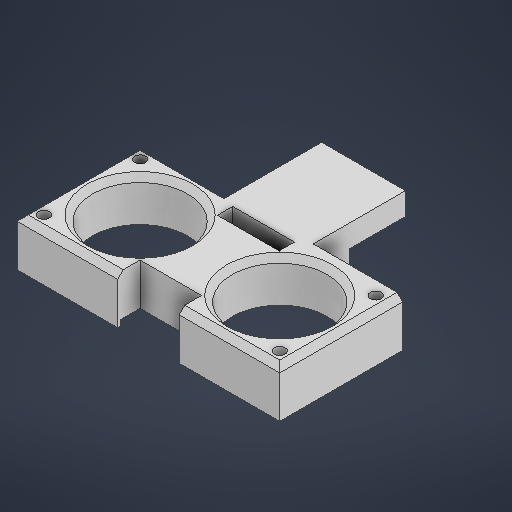
# Autodesk Inventor part: us-sensor-mount
Saved by Autodesk Inventor 2026.2 (Build 302298010, 298A)
## iProperties
Created: 2026-02-26
Part Number: us-sensor-mount
Material: Generic
Document SubType Name: Modeling
Designer: dm2166
Density: 1 g/cm^3
Appearance: Default
Author: dm2166
Autodesk Inventor part; units mm, degrees
ref_plane "YZ Plane" through (0, 0, 0) normal (1, 0, 0) x (0, 1, 0)
ref_plane "XZ Plane" through (0, 0, 0) normal (0, 1, 0) x (-1, 0, 0)
ref_plane "XY Plane" through (0, 0, 0) normal (0, 0, 1) x (1, 0, 0)
sketch "Sketch1" plane through (0, 0, 0) normal (0, 1, 0) x (-1, 0, 0)
  circle A0 centre (-15.215, 10.4919) radius 8.5
  circle A1 centre (9.785, 10.4919) radius 8.5
  line L0 (-2.515, 3.3319) -> (-2.515, 1.1919)
  line L1 (-0.375, 3.3319) -> (-2.515, 3.3319)
  line L2 (-0.375, 1.1919) -> (-0.375, 3.3319)
  line L3 (-2.515, 1.1919) -> (-0.375, 1.1919)
  line L4 (-5.455, 3.3319) -> (-7.595, 3.3319)
  line L5 (-5.455, 1.1919) -> (-5.455, 3.3319)
  line L6 (-7.595, 1.1919) -> (-5.455, 1.1919)
  line L7 (-7.595, 3.3319) -> (-7.595, 1.1919)
  circle A2 centre (-23.815, 19.0919) radius 1
  circle A3 centre (-23.815, 1.8919) radius 1
  circle A4 centre (18.385, 1.8919) radius 1
  circle A5 centre (18.385, 19.0919) radius 1
  line L8 (-25.215, 20.4919) -> (-25.215, 0.4919)
  line L9 (-25.215, 0.4919) -> (19.785, 0.4919)
  line L10 (19.785, 0.4919) -> (19.785, 20.4919)
  line L11 (19.785, 20.4919) -> (-25.215, 20.4919)
  line L12 (-2.915, 3.3319) -> (-5.055, 3.3319)
  line L13 (-2.915, 1.1919) -> (-2.915, 3.3319)
  line L14 (-5.055, 1.1919) -> (-2.915, 1.1919)
  line L15 (-5.055, 3.3319) -> (-5.055, 1.1919)
  line L16 (2.165, 3.3319) -> (0.025, 3.3319)
  line L17 (2.165, 1.1919) -> (2.165, 3.3319)
  line L18 (0.025, 1.1919) -> (2.165, 1.1919)
  line L19 (0.025, 3.3319) -> (0.025, 1.1919)
  line L20 (-8.2373, 3.6319) -> (2.8072, 3.6319)
  line L21 (2.8072, 3.6319) -> (2.8072, 0.8919)
  line L22 (2.8072, 0.8919) -> (-8.2373, 0.8919)
  line L23 (-8.2373, 0.8919) -> (-8.2373, 3.6319)
  line L24 (-8.2373, 3.6319) -> (2.8072, 0.8919) construction
  line L25 (2.8072, 3.6319) -> (-8.2373, 0.8919) construction
  line L26 (-10.215, 17.9919) -> (4.785, 17.9919)
  line L27 (4.785, 17.9919) -> (4.785, -17.0081)
  line L28 (4.785, -17.0081) -> (-10.215, -17.0081)
  line L29 (-10.215, -17.0081) -> (-10.215, 17.9919)
  line L30 (-10.215, 17.9919) -> (4.785, -17.0081) construction
  line L31 (4.785, 17.9919) -> (-10.215, -17.0081) construction
  line L32 (-10.215, -17.0081) -> (4.785, -17.0081)
  line L33 (4.785, -17.0081) -> (4.785, -7.0081)
  line L34 (4.785, -7.0081) -> (-10.215, -7.0081)
  line L35 (-10.215, -7.0081) -> (-10.215, -17.0081)
  line L36 (-26.215, 21.4919) -> (20.785, 21.4919)
  line L37 (20.785, 21.4919) -> (20.785, -0.5081)
  line L38 (20.785, -0.5081) -> (-26.215, -0.5081)
  line L39 (-26.215, -0.5081) -> (-26.215, 21.4919)
  line L40 (-26.215, 21.4919) -> (20.785, -0.5081) construction
  line L41 (20.785, 21.4919) -> (-26.215, -0.5081) construction
  line L42 (20.285, 20.9919) -> (-25.715, 20.9919)
  line L43 (-25.715, 20.9919) -> (-25.715, -0.0081)
  line L44 (-25.715, -0.0081) -> (20.285, -0.0081)
  line L45 (20.285, -0.0081) -> (20.285, 20.9919)
  line L46 (20.285, 20.9919) -> (-25.715, -0.0081) construction
  line L47 (-25.715, 20.9919) -> (20.285, -0.0081) construction
  line L48 (4.785, -0.0081) -> (5.285, -0.0081)
  line L49 (5.285, -0.0081) -> (5.285, -0.5081)
  line L50 (-10.215, -0.0081) -> (-10.415, -0.0081)
  line L51 (-10.215, -0.0081) -> (-10.415, -0.0081)
  line L52 (-10.215, -0.5081) -> (-11.215, -0.5081)
  line L53 (-10.2622, -0.5234) -> (-10.7622, -0.5234)
  line L54 (-10.7622, -0.5234) -> (-10.7622, -0.0081)
  line L55 (2.785, 21.4919) -> (-8.215, 21.4919)
  line L56 (-8.215, 21.4919) -> (-8.215, 17.4919)
  line L57 (-8.215, 17.4919) -> (2.785, 17.4919)
  line L58 (2.785, 17.4919) -> (2.785, 21.4919)
  point P0 (0, 0)
  point P1 (-2.715, 10.4919)
  point P2 (-2.715, 2.2619)
  point P3 (-2.715, 0.4919)
  point P4 (4.785, -0.5081)
  point P5 (-10.7622, -0.5081)
  point P6 (-8.215, 21.4919)
  dimension "d0" = 15
  dimension "d1" = 35
  dimension "d2" = 10
  dimension "d3" = 47
  dimension "d4" = 22
  dimension "d5" = 17
  dimension "d6" = 17
  dimension "d11" = 20
  dimension "d12" = 45
  dimension "d13" = 46
  dimension "d14" = 21
  dimension "d15" = 0.5
  dimension "d19" = 0.5
  dimension "d27" = 17
  dimension "d28" = 17
  dimension "d29" = 4
  constraints: 118 end point, 13 point on line, 12 parallel, 9 midpoint, 8 perpendicular, 7 horizontal, 6 centre point, 1 collinear
  measures "d0" distance of L27.end L28.end
  measures "d1" distance of L28.end L26.start
  measures "d2" distance of L33.end L32.end
  measures "d3" distance of L37.end L38.end
  measures "d4" distance of L36.end L37.end
  measures "d5" diameter of A1
  measures "d6" diameter of A0
  measures "d11" distance of L9.end L10.end
  measures "d12" distance of L10.end L8.start
  measures "d13" distance of L44.end L43.end
  measures "d14" distance of L43.end L42.end
  measures "d15" distance of L48.start L48.end
  measures "d19" distance of L53.start L53.end
  measures "d27" distance between parallel lines of L10 L58
  measures "d28" distance between parallel lines of L8 L56
  measures "d29" distance of L57.end L55.start
extrude "Extrusion1" add sketch "Sketch1" along normal blind 7.5 contours A0 L29 L26 L56 L57 L58 L27 A1 L9 | A0 L29 L9 L8 L11 L56 L26 | L29 L44 L43 L42 L56 L11 L8 L9 | L9 L27 L44 L29 | L56 L11 L58 L26 | L26 L58 L57 L56 | L27 A1 L26 L58 L11 L10 L9 | L9 L10 L11 L58 L42 L45 L44 L27 | L44 L27 L38 L29 | L29 L38 L54 L44 | L56 L42 L58 L11 | L44 L49 L38 L27 | L38 L27 L34 L29 | L56 L36 L58 L42 | L42 L43 L44 L54 L38 L39 L36 L56 | L44 L45 L42 L58 L36 L37 L38 L49
extrude "Extrusion2" add sketch "Sketch1" along normal blind 7.5 contours L34 L27 L28 L29
extrude "Extrusion3" add sketch "Sketch1" against normal blind 1 contours L56 L36 L58 L42 | L42 L43 L44 L54 L38 L39 L36 L56 | L44 L45 L42 L58 L36 L37 L38 L49
chamfer "Chamfer1" distance 1 angle 45 6 edges at (-20.785, 7.5, 10.4919) (-12.785, 7.5, -0.5081) (2.715, 7.5, 21.4919) (26.215, 7.5, 10.4919) (23.715, 7.5, 10.4919) (-1.285, 7.5, 10.4919)
extrude "Extrusion4" cut sketch "Sketch1" along normal blind 3.5 contours L34 L27 L28 L29
extrude "Extrusion5" cut sketch "Sketch1" along normal blind 7.5 and the other way blind 1.75 contours L56 L11 L58 L26 | L26 L58 L57 L56 | L56 L42 L58 L11 | L56 L36 L58 L42
body "Solid1"
